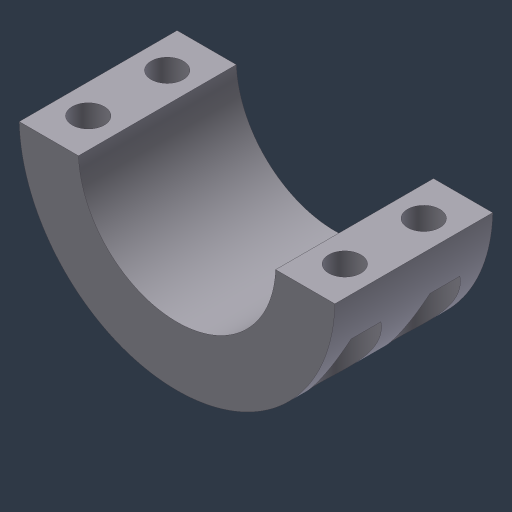
# Autodesk Inventor part: TOP,BEARING_BLOCK,ELEVATOR
Saved by Autodesk Inventor 2024.3 (Build 283343000, 343)
## iProperties
Category: _
Manager: _
ILogicPurgeVersion: 0.0.0.0
OnSaveVersion: 2.2.20.20
Created: 2025-03-05
Part Number: TOP,BEARING_BLOCK,ELEVATOR
Checked By: 00
Engr Approved By: _
User Status: Work In Process
Material: Aluminum, 7075-T6
Description: STANDARD (mm)
Document SubType Name: Modeling
Mfg Approved By: Stephen.Oerton
Designer: John Thibert
Manufacturer: Standard
Standards Organization: Custom
Density: 2.81 g/cm^3
Appearance: Metal-AL-6061 (Flat)
CN_MASS: 0.0
CN_SERVICEABLE: _
FIRST_DESCRIPTION: _
SECOND_DESCRIPTION: _
THIRD_DESCRIPTION: _
ModelCat: Uncategorized
Subject: _
Author: John Thibert
Keywords: -
Revision Number: A
Autodesk Inventor part; units mm, degrees
ref_plane "YZ Plane" through (0, 0, 0) normal (1, 0, 0) x (0, 1, 0)
ref_plane "XZ Plane" through (0, 0, 0) normal (0, 1, 0) x (-1, 0, 0)
ref_plane "XY Plane" through (0, 0, 0) normal (0, 0, 1) x (1, 0, 0)
sketch "Sketch2" plane through (0, 0, 0) normal (0, 0, 1) x (1, 0, 0)
  arc A0 (-25.3921, -0.635) -> (25.3921, -0.635) centre (0, 0) ccw
  line L0 (25.3921, -0.635) -> (-25.3921, -0.635)
  line L1 (-35.5489, 0) -> (35.5489, 0) construction
  dimension "d0" = 25.4
  dimension "d1" = 0.635
  constraints: 2 end point, 2 point on circle, 1 centre point, 1 coincident, 1 horizontal
  measures "d0" radius of A0
  measures "d1" distance between parallel lines of L0 L1
extrude "Extrusion1" add sketch "Sketch2" along normal mid plane 25.4
sketch "Sketch3" plane through (0, 0, 12.7) normal (0, 0, 1) x (1, 0, 0)
  point P0 (0, 0)
  point P1 (0, 0)
  constraints: 1 coincident
hole "Hole1" at (0, 0, 12.7) direction (0, 0, -1) diameter 31.75 end through all
ref_plane "Work Plane1" through (25.3921, -13.335, 12.7) normal (0, 1, 0) x (1, 0, 0)
sketch "Sketch4" plane through (25.3921, -13.335, 12.7) normal (0, 1, 0) x (1, 0, 0)
  line L0 (-46.0296, 6.35) -> (-4.7546, 6.35) construction
  line L1 (-4.7546, 6.35) -> (-4.7546, 19.05) construction
  line L2 (-4.7546, 19.05) -> (-46.0296, 19.05) construction
  line L3 (-46.0296, 19.05) -> (-46.0296, 6.35) construction
  line L4 (-46.0296, 6.35) -> (-4.7546, 19.05) construction
  line L5 (-4.7546, 6.35) -> (-46.0296, 19.05) construction
  point P0 (-25.3921, 12.7)
  dimension "d13" = 41.275
  dimension "d14" = 12.7
  constraints: 12 end point, 4 coincident, 2 midpoint, 2 parallel, 1 horizontal, 1 perpendicular
  measures "d13" distance of L2.end L1.end
  measures "d14" distance of L1.end L0.end
hole "Hole2" at (20.6375, -13.335, -6.35) at (20.6375, -13.335, 6.35) at (-20.6375, -13.335, -6.35) at (-20.6375, -13.335, 6.35) direction (0, 1, 0) diameter 5.1562 depth 13.6144 tip angle 118 start extended yes counterbore diameter 8.3312 counterbore depth 5.1562 clearance for "Socket Head Cap Screw" size "#10" standard "(CL)Ansi Unified Screw Threads"
body "Solid1"
